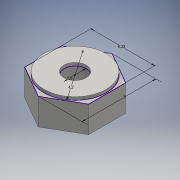
# Autodesk Inventor part: ナット
Saved by Autodesk Inventor 2016 (Build 200138000, 138)
## iProperties
Created: 2016-12-02
Part Number: ナット
Material: 一般
Document SubType Name: Modeling
Designer: KOTA-NPC2
Density: 1 g/cm^3
Appearance: 既定
Author: KOTA-NPC2
Autodesk Inventor part; units mm, degrees
ref_plane "YZ Plane" through (0, 0, 0) normal (1, 0, 0) x (0, 1, 0)
ref_plane "XZ Plane" through (0, 0, 0) normal (0, 1, 0) x (-1, 0, 0)
ref_plane "XY Plane" through (0, 0, 0) normal (0, 0, 1) x (1, 0, 0)
sketch "スケッチ1" plane through (0, 0, 0) normal (0, 0, 1) x (1, 0, 0)
  line L0 (0, -2.5) -> (-2.1651, -1.25)
  line L1 (-2.1651, -1.25) -> (-2.1651, 1.25)
  line L2 (-2.1651, 1.25) -> (0, 2.5)
  line L3 (0, 2.5) -> (2.1651, 1.25)
  line L4 (2.1651, 1.25) -> (2.1651, -1.25)
  line L5 (2.1651, -1.25) -> (0, -2.5)
  circle A0 centre (0, 0) radius 0.75
  circle A1 centre (0, 0) radius 2.1
  dimension "d0" = 5
  dimension "d1" = 4.3301
  dimension "d2" = 1.5
  dimension "d3" = 4.2
  constraints: 12 end point, 3 coincident, 2 centre point, 13 other
  measures "d0" distance of L0.start L2.end
  measures "d1" horizontal distance of L0.end L3.end
  measures "d2" diameter of A0
  measures "d3" diameter of A1
extrude "押し出し1" add sketch "スケッチ1" against normal blind 1.8 contours L0 L1 L2 L3 L4 L5 | A1
extrude "押し出し2" add sketch "スケッチ1" along normal blind 0.2 contours A1
